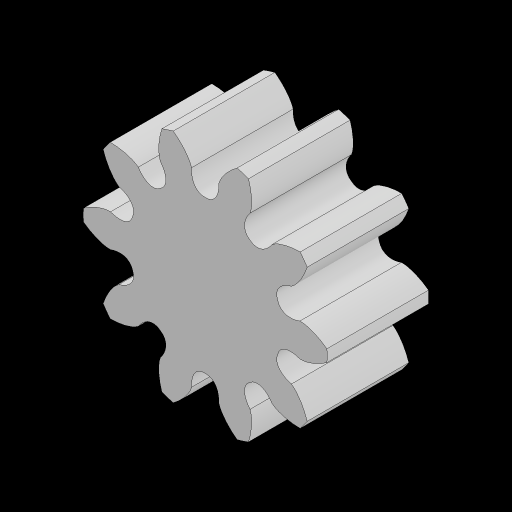
# Autodesk Inventor part: Intermediate Gear
Saved by Autodesk Inventor 2023.2 (Build 272271030, 271C)
## iProperties
Created: 2023-11-17
Part Number: Intermediate Gear
Material: Generic
Document SubType Name: Modeling
Designer: robpl
Density: 1 g/cm^3
Appearance: Default
Author: robpl
Autodesk Inventor part; units mm, degrees
ref_plane "YZ Plane" through (0, 0, 0) normal (1, 0, 0) x (0, 1, 0)
ref_plane "XZ Plane" through (0, 0, 0) normal (0, 1, 0) x (-1, 0, 0)
ref_plane "XY Plane" through (0, 0, 0) normal (0, 0, 1) x (1, 0, 0)
sketch "Sketch1" plane through (0, 0, 0) normal (0, 0, 1) x (1, 0, 0)
  spline S0 degree 3 poles (-1.5724, 5.7903) (-1.5241, 5.7538) (-1.4275, 5.6808) (-1.2901, 5.5617) (-1.1591, 5.4358) (-1.0361, 5.3018) (-0.9225, 5.1599) (-0.8373, 5.0346) (-0.7763, 4.9299) (-0.7351, 4.8489) (-0.6983, 4.7657) (-0.6806, 4.7078) (-0.6718, 4.6788) knots 0 0 0 0 0.018166 0.036332 0.054498 0.072663 0.090828 0.10899 0.118074 0.127157 0.136239 0.145318 0.145318 0.145318 0.145318
  spline S1 degree 3 poles (-0.6718, 4.6788) (-0.6728, 4.6515) (-0.6747, 4.5969) (-0.6727, 4.5149) (-0.6661, 4.4332) (-0.6531, 4.3522) (-0.6372, 4.2718) (-0.6127, 4.1935) (-0.583, 4.117) (-0.5457, 4.0439) (-0.5003, 3.9755) (-0.4473, 3.9128) (-0.3863, 3.8577) (-0.3175, 3.8127) (-0.2431, 3.7778) (-0.1769, 3.7601) (-0.1229, 3.7512) (-0.0683, 3.7492) (0, 3.7505) (0.0683, 3.7492) (0.1229, 3.7512) (0.1769, 3.7601) (0.2431, 3.7778) (0.3175, 3.8127) (0.3863, 3.8577) (0.4473, 3.9128) (0.5003, 3.9755) (0.5457, 4.0439) (0.583, 4.117) (0.6127, 4.1935) (0.6372, 4.2718) (0.6531, 4.3522) (0.6661, 4.4332) (0.6727, 4.5149) (0.6747, 4.5969) (0.6728, 4.6515) (0.6718, 4.6788) knots 0 0 0 0 0.008194 0.016389 0.024583 0.032776 0.040969 0.049163 0.057354 0.065548 0.073742 0.081932 0.090121 0.098308 0.106495 0.114678 0.118776 0.122873 0.131067 0.139261 0.143358 0.147456 0.155639 0.163826 0.172012 0.180202 0.188392 0.196585 0.204779 0.212971 0.221165 0.229358 0.237551 0.245745 0.253939 0.262134 0.262134 0.262134 0.262134
  spline S2 degree 3 poles (0.6718, 4.6788) (0.6806, 4.7078) (0.6983, 4.7657) (0.7351, 4.8489) (0.7763, 4.9299) (0.8373, 5.0346) (0.9225, 5.1599) (1.0361, 5.3018) (1.1591, 5.4358) (1.2901, 5.5617) (1.4275, 5.6808) (1.5241, 5.7538) (1.5724, 5.7903) knots 0 0 0 0 0.009079 0.018161 0.027244 0.036327 0.05449 0.072655 0.09082 0.108986 0.127152 0.145318 0.145318 0.145318 0.145318
  circle A0 centre (0, 0) radius 3.75 construction
  circle A1 centre (0, 0) radius 4.6985 construction
  circle A2 centre (0, 0) radius 5 construction
  circle A3 centre (0, 0) radius 6
  point P0 (-1.4287, 5.6792)
  point P1 (-1.2911, 5.5606)
  point P2 (-1.1604, 5.4344)
  point P3 (-1.0377, 5.3005)
  point P4 (-0.9244, 5.1585)
  point P5 (-0.8227, 5.0081)
  point P6 (-0.7771, 4.9295)
  point P7 (-0.7358, 4.8486)
  point P8 (-0.7, 4.7651)
  point P9 (-0.6739, 4.5969)
  point P10 (-0.6719, 4.515)
  point P11 (-0.665, 4.4333)
  point P12 (-0.6526, 4.3523)
  point P13 (-0.6357, 4.2722)
  point P14 (-0.6118, 4.1938)
  point P15 (-0.5817, 4.1176)
  point P16 (-0.5443, 4.0447)
  point P17 (-0.499, 3.9764)
  point P18 (-0.4459, 3.914)
  point P19 (-0.385, 3.8594)
  point P20 (-0.3166, 3.8144)
  point P21 (-0.2422, 3.7801)
  point P22 (-0.1634, 3.7583)
  point P23 (-0.1229, 3.752)
  point P24 (-0.0819, 3.7499)
  point P25 (0, 3.75)
  point P26 (0.0819, 3.7499)
  point P27 (0.1229, 3.752)
  point P28 (0.1634, 3.7583)
  point P29 (0.2422, 3.7801)
  point P30 (0.3166, 3.8144)
  point P31 (0.385, 3.8594)
  point P32 (0.4459, 3.914)
  point P33 (0.499, 3.9764)
  point P34 (0.5443, 4.0447)
  point P35 (0.5817, 4.1176)
  point P36 (0.6118, 4.1938)
  point P37 (0.6357, 4.2722)
  point P38 (0.6526, 4.3523)
  point P39 (0.665, 4.4333)
  point P40 (0.6719, 4.515)
  point P41 (0.6739, 4.5969)
  point P42 (0.7, 4.7651)
  point P43 (0.7358, 4.8486)
  point P44 (0.7771, 4.9295)
  point P45 (0.8227, 5.0081)
  point P46 (0.9244, 5.1585)
  point P47 (1.0377, 5.3005)
  point P48 (1.1604, 5.4344)
  point P49 (1.2911, 5.5606)
  point P50 (1.4287, 5.6792)
  constraints: 4 centre point, 2 point on circle, 117 other
extrude "Extrusion1" add sketch "Sketch1" against normal blind 5
extrude "Extrusion2" cut sketch "Sketch1" against normal through all contours A3 S2 S1 S0 picked at (0.1835, 5.2736)
pattern_circular "Circular Pattern1" count 10 over 360 about axis through (0, 0, 0) along (0, 0, -1) of "Extrusion2"
equation "\"Module\" = 1"
equation "\"PressureAngle\" = 20deg"
equation "\"UnitProfileClearance\" = 0.25"
equation "\"UnitRoundRadius\" = 0.35"
equation "\"HeadDiameter\" = 12"
equation "\"RootDiameter\" = 7.5"
equation "\"BaseDiameter\" = 9.39693"
equation "\"HelixAngle\" = 0"
equation "\"UnitCorrection\" = 0"
equation "\"UnitAddendumModification\" = 0"
equation "\"CircularPitch\" = 3.141593"
equation "\"UnitBacklashShift\" = 0"
equation "\"TotalToolShift\" = 0"
equation "\"IsInternal\" = 0"
body "Solid1"
